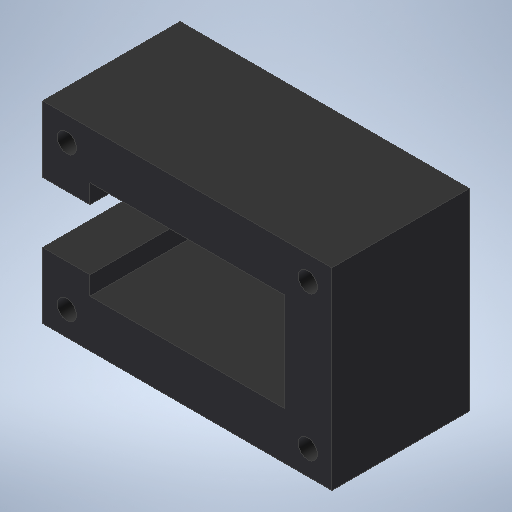
# Autodesk Inventor part: Servoholder
Saved by Autodesk Inventor 2025 (Build 290162000, 162)
## iProperties
Created: 2025-12-03
Part Number: Servoholder
Material: Generic
Document SubType Name: Modeling
Designer: ruven
Density: 1 g/cm^3
Appearance: Default
Author: ruven
Autodesk Inventor part; units mm, degrees
ref_plane "YZ Plane" through (0, 0, 0) normal (1, 0, 0) x (0, 1, 0)
ref_plane "XZ Plane" through (0, 0, 0) normal (0, 1, 0) x (-1, 0, 0)
ref_plane "XY Plane" through (0, 0, 0) normal (0, 0, 1) x (1, 0, 0)
sketch "Sketch1" plane through (0, 0, 0) normal (0, 1, 0) x (-1, 0, 0)
  line L0 (-20.2, -10.2) -> (20.2, -10.2)
  line L1 (20.2, -10.2) -> (20.2, 10.2)
  line L2 (20.2, 10.2) -> (-20.2, 10.2)
  line L3 (-20.2, 10.2) -> (-20.2, -10.2)
  line L4 (-20.2, -10.2) -> (20.2, 10.2) construction
  line L5 (20.2, -10.2) -> (-20.2, 10.2) construction
  line L6 (-30, -20) -> (30, -20)
  line L7 (30, -20) -> (30, 20)
  line L8 (30, 20) -> (-30, 20)
  line L9 (-30, 20) -> (-30, -20)
  line L10 (-30, -20) -> (30, 20) construction
  line L11 (30, -20) -> (-30, 20) construction
  circle A0 centre (25, 15) radius 2
  circle A1 centre (25, -15) radius 2
  circle A2 centre (-25, 15) radius 2
  circle A3 centre (-25, -15) radius 2
  point P0 (0, 0)
  dimension "d0" = 20.4
  dimension "d1" = 40.4
  dimension "d2" = 60
  dimension "d3" = 40
  dimension "d4" = 4
  dimension "d5" = 4
  dimension "d7" = 4
  dimension "d8" = 5
  dimension "d9" = 5
  dimension "d10" = 5
  dimension "d11" = 5
  dimension "d13" = 4
  dimension "d14" = 5
  dimension "d15" = 5
  dimension "d16" = 5
  dimension "d17" = 5
  constraints: 24 end point, 4 centre point, 4 midpoint, 4 parallel, 2 horizontal, 2 perpendicular
  measures "d0" distance of L0.end L1.end
  measures "d1" distance of L1.end L2.end
  measures "d2" distance of L7.end L8.end
  measures "d3" distance between parallel lines of L6 L8
  measures "d4" diameter of A0
  measures "d5" diameter of A1
  measures "d7" diameter of A2
  measures "d8" distance from line of L7 A0.centre
  measures "d9" distance from line of L8 A0.centre
  measures "d10" distance from line of L7 A1.centre
  measures "d11" distance from line of L6 A1.centre
  measures "d13" diameter of A3
  measures "d14" distance from line of L6 A3.centre
  measures "d15" distance from line of L9 A3.centre
  measures "d16" distance from line of L9 A2.centre
  measures "d17" distance from line of L8 A2.centre
extrude "Extrusion1" add sketch "Sketch1" along normal blind 28.5
sketch "Sketch2" plane through (0, 28.5, 0) normal (0, 1, 0) x (1, 0, 0)
  circle A0 centre (-24.25, -4.75) radius 1.5
  circle A1 centre (-24.25, 4.75) radius 1.5
  circle A2 centre (24.25, -4.75) radius 1.5
  circle A3 centre (24.25, 4.75) radius 1.5
  line L0 (20.2, 10.2) -> (20.2, -10.2) projected
  point P0 (0, 0)
  point P1 (20.2, 0)
  dimension "d20" = 3
  dimension "d21" = 3
  dimension "d22" = 3
  dimension "d23" = 3
  dimension "d24" = 48.5
  dimension "d25" = 24.25
  dimension "d26" = 48.5
  dimension "d27" = 24.25
  dimension "d28" = 9.5
  dimension "d29" = 4.75
  dimension "d30" = 9.5
  dimension "d31" = 4.75
  constraints: 4 centre point, 1 midpoint
  measures "d20" diameter of A0
  measures "d21" diameter of A1
  measures "d22" diameter of A3
  measures "d23" diameter of A2
  measures "d24" distance of A2.centre A0.centre
  measures "d25" horizontal distance of point (0, 0) A2.centre
  measures "d26" distance of A1.centre A3.centre
  measures "d27" horizontal distance of point (0, 0) A1.centre
  measures "d28" distance of A1.centre A0.centre
  measures "d29" vertical distance of point (0, 0) A0.centre
  measures "d30" distance of A3.centre A2.centre
  measures "d31" vertical distance of point (20.2, 0) A3.centre
extrude "Extrusion2" cut sketch "Sketch2" against normal blind 20
sketch "Sketch3" plane through (0, 28.5, 0) normal (0, 1, 0) x (1, 0, 0)
  line L0 (-30, 20) -> (-30, -20) projected
  line L1 (-20.2, -10.2) -> (-20.2, 10.2) projected
  line L2 (-30, 6.3495) -> (-20.2, 6.3495)
  line L3 (-20.2, 6.3495) -> (-20.2, -6.2601)
  line L4 (-20.2, -6.2601) -> (-30, -6.2601)
  line L5 (-30, -6.2601) -> (-30, 6.3495)
  point P0 (0, 0)
  point P1 (-20.2, 6.3495)
  constraints: 8 end point, 2 parallel, 2 point on line, 1 horizontal, 1 perpendicular
extrude "Extrusion3" cut sketch "Sketch3" against normal through all
body "Solid1"
